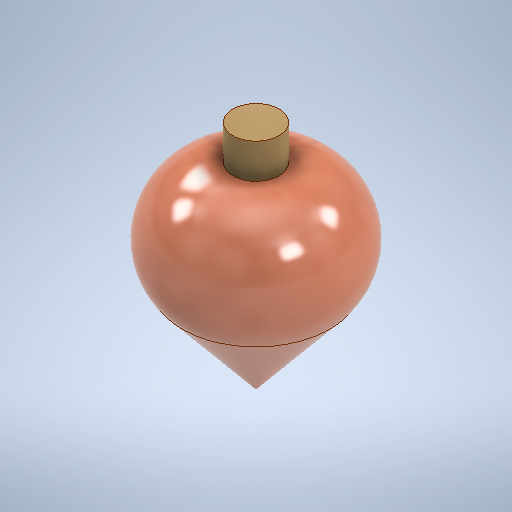
# Autodesk Inventor part: peca_003_001
Saved by Autodesk Inventor 2025.2 (Build 292293000, 293)
## iProperties
Created: 2025-03-25
Part Number: peca_003_001
Material: Madeira (Nogueira)
Document SubType Name: Modeling
Designer: Carlos Dias
Density: 0.55 g/cm^3
Appearance: Nogueira - Natural polido
Author: Carlos Dias
Autodesk Inventor part; units mm, degrees
ref_plane "YZ Plane" through (0, 0, 0) normal (1, 0, 0) x (0, 1, 0)
ref_plane "XZ Plane" through (0, 0, 0) normal (0, 1, 0) x (-1, 0, 0)
ref_plane "XY Plane" through (0, 0, 0) normal (0, 0, 1) x (1, 0, 0)
sketch "Esboço1" plane through (0, 0, 0) normal (0, 0, 1) x (1, 0, 0)
  line L0 (-2, 20) -> (0, 20)
  arc A0 (-2, 17) -> (-6.3739, 7.7054) centre (-2, 11.3235) ccw
  line L1 (-6.3739, 7.7054) -> (0, 0)
  line L2 (-2, 20) -> (-2, 17)
  line L3 (0, 20) -> (0, 0)
  line L4 (0, -4) -> (0, 24) projected
  dimension "d0" = 2
  dimension "d1" = 20
  dimension "d2" = 10
  dimension "d3" = 3
  constraints: 8 end point, 2 point on circle, 2 vertical, 1 centre point, 1 coincident, 1 horizontal, 1 line through centre, 1 tangent, 1 vertical alignment
  measures "d0" distance of L0.start L0.end
  measures "d1" distance from line of point (0, 0) L0
  measures "d2" distance of L1.start L1.end
  measures "d3" distance of L0.start L2.end
revolve "Revolução1" add sketch "Esboço1" angle 360 about axis through (0, -10, 0) along (0, 1, 0)
